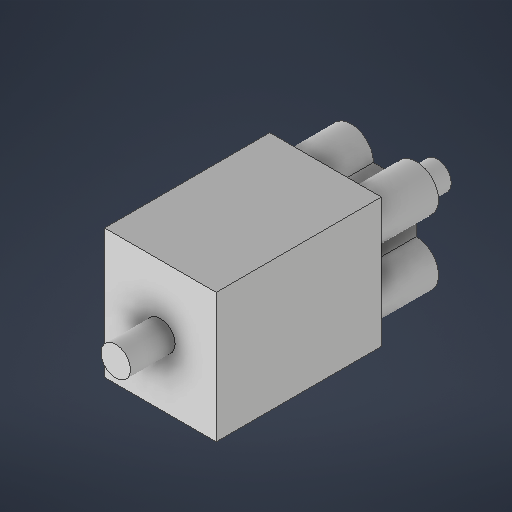
# Autodesk Inventor part: Adafruit_1528-4663-ND
Saved by Autodesk Inventor 2026.2 (Build 302298000, 298)
## iProperties
Created: 2026-01-28
Part Number: Adafruit_1528-4663-ND
Material: Generic
Document SubType Name: Modeling
Designer: vckot
Density: 1 g/cm^3
Appearance: Default
Author: vckot
Autodesk Inventor part; units mm, degrees
ref_plane "YZ Plane" through (0, 0, 0) normal (1, 0, 0) x (0, 1, 0)
ref_plane "XZ Plane" through (0, 0, 0) normal (0, 1, 0) x (-1, 0, 0)
sketch "Sketch1" plane through (0, 0, 0) normal (0, 0, 1) x (1, 0, 0)
  line L0 (0, 0) -> (12.5, 0)
  line L1 (12.5, 0) -> (12.5, 14.5)
  line L2 (12.5, 14.5) -> (0, 14.5)
  line L3 (0, 14.5) -> (0, 0)
  dimension "d0" = 14.5
  dimension "d1" = 12.5
  constraints: 8 end point, 2 parallel, 1 horizontal, 1 perpendicular
  measures "d0" distance of L0.end L1.end
  measures "d1" distance of L1.end L2.end
extrude "Extrusion1" add sketch "Sketch1" against normal blind 18.5
sketch "Sketch2" plane through (0, 0, -18.5) normal (0, 0, -1) x (-1, 0, 0)
  circle A0 centre (-9.9, 3.6) radius 2.5
  circle A1 centre (-2.6, 3.6) radius 2.5
  circle A2 centre (-2.6, 10.9) radius 2.5
  circle A3 centre (-9.9, 10.9) radius 2.5
  line L0 (-9.9, 10.9) -> (-9.9, 3.6) construction
  line L1 (-12.5, 14.5) -> (-12.5, 0) construction
  line L2 (-9.9, 10.9) -> (-2.6, 10.9) construction
  line L3 (0, 14.5) -> (-12.5, 14.5) construction
  line L4 (-7.4, 10.9) -> (-5.1, 10.9)
  line L5 (-2.6, 8.4) -> (-2.6, 6.1)
  line L6 (-7.4, 3.6) -> (-5.1, 3.6)
  line L7 (-9.9, 8.4) -> (-9.9, 6.1)
  circle A4 centre (-9.9, 10.9) radius 1.75
  circle A5 centre (-2.6, 10.9) radius 1.75
  circle A6 centre (-2.6, 3.6) radius 1.75
  circle A7 centre (-9.9, 3.6) radius 1.75
  circle A8 centre (-6.25, 7.25) radius 1.57
  point P0 (0, 0)
  point P1 (-9.9, 7.25)
  point P2 (-12.5, 7.25)
  point P3 (-6.25, 10.9)
  point P4 (-6.25, 14.5)
  point P5 (-6.25, 3.6)
  point P6 (-2.6, 7.25)
  dimension "d4" = 5
  dimension "d5" = 12.3
  dimension "d6" = 7.3
  dimension "d7" = 0.75
  dimension "d8" = 3.14
  constraints: 12 end point, 9 centre point, 8 point on circle, 6 equal radius, 6 midpoint, 4 coincident, 4 horizontal alignment, 4 point on line, 4 vertical alignment, 2 perpendicular, 1 horizontal, 1 vertical
  measures "d4" diameter of A3
  measures "d6" distance of L2.end L0.start
  measures "d7" radial gap between concentric circles of A3 A4
  measures "d8" diameter of A8
sketch "Sketch3" plane through (0, 0, 0) normal (0, 0, 1) x (1, 0, 0)
  circle A0 centre (6.25, 7.1995) radius 1.65
  point P0 (0, 0)
  dimension "d9" = 3.3
  constraints: 1 centre point
  measures "d9" diameter of A0
extrude "Extrusion2" add sketch "Sketch3" along normal blind 5
extrude "Extrusion3" add sketch "Sketch2" along normal blind 6.52
extrude "Extrusion4" add sketch "Sketch2" along normal blind 12.52 contours A8
ref_plane "Work Plane1" through (6.25, 0, 0) normal (1, 0, 0) x (0, 0, -1)
sketch "Sketch4" plane through (6.25, 0, 0) normal (1, 0, 0) x (0, 0, -1)
  line L0 (18.5, 10.9) -> (25.02, 10.9) projected
  line L1 (21.76, 10.9) -> (23.385, 10.9)
  line L2 (23.385, 10.9) -> (23.385, 14.1)
  line L3 (23.385, 18.1) -> (21.76, 18.1)
  line L4 (21.76, 18.1) -> (21.76, 10.9)
  line L5 (21.76, 10.9) -> (23.385, 10.9)
  line L6 (23.385, 10.9) -> (23.385, 14.1)
  line L7 (21.76, 18.1) -> (21.76, 15.1)
  line L8 (23.6683, 15.1) -> (23.81, 15.1)
  line L9 (23.81, 15.1) -> (23.385, 18.1)
  line L10 (21.76, 18.1) -> (21.76, 14.1)
  line L11 (23.385, 14.1) -> (23.81, 14.1)
  line L12 (23.81, 14.1) -> (23.6683, 15.1)
  point P0 (0, 0)
  dimension "d16" = 1.625
  dimension "d17" = 7.2
  dimension "d18" = 90
  dimension "d19" = 3
  dimension "d20" = 2.05
  dimension "d21" = 4
  dimension "d22" = 1.625
  dimension "d23" = 2.05
  dimension "d24" = 3
  constraints: 24 end point, 4 perpendicular, 3 parallel, 3 point on line, 1 horizontal, 1 midpoint, 1 vertical alignment
  measures "d16" distance of L1.start L1.end
  measures "d17" distance of L1.end L3.start
  measures "d18" angle of L2 L1
  measures "d19" distance of L3.end L7.end
  measures "d20" distance of L7.end L8.end
  measures "d21" distance of L3.end L10.end
  measures "d22" distance of L3.start L3.end
  measures "d23" distance of L10.end L11.end
  measures "d24" distance between parallel lines of L8 L3
revolve "Revolution1" add sketch "Sketch4" angle 360 about axis through (6.25, 18.1, -21.76) along (0, -1, 0)
pattern_circular "Circular Pattern1" count 4 over 360 about axis through (6.25, 7.25, -18.5) along (0, 0, -1) of "Revolution1"
delete faces "Delete Face1" heal yes whole lump no faces at (8.0785, 15.7667, -22.4534) (5.7435, 18.1, -22.5272) (8.079, 14.2111, -22.6505) (7.3088, 12.1519, -20.5273) (6.0865, 14.1, -23.6485) (6.0865, 15.1, -23.7429) (14.7667, 7.718, -23.6587) (14.1, 6.0575, -23.3527) (13.2111, 5.421, -22.6505) (13.1, 7.4135, -23.6485) (11.1519, 6.1912, -20.5273) (17.1, 7.7565, -22.5272) (6.718, -1.2667, -23.6587) (4.421, 0.2889, -22.6505) (5.0575, -0.6, -23.3527) (6.4135, 0.4, -23.6485) (5.1912, 2.3481, -20.5273) (6.7565, -3.6, -22.5272)
body "Solid1"
